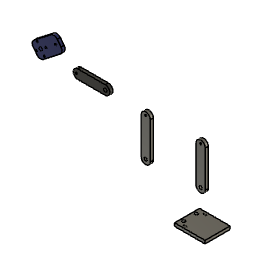
laserCut v11 (Autodesk Fusion 360 design; units mm, degrees)
Autodesk Fusion 360 part; units mm, degrees
sketch "Sketch19" plane through (0, 0, 0) normal (0, 1, 0) x (1, 0, 0)
  line L0 (-204.4398, 88.4329) -> (-125.5431, 26.9894)
  line L1 (-125.5431, 26.9894) -> (-94.8213, 66.4377)
  line L2 (-94.8213, 66.4377) -> (-173.7181, 127.8812)
  line L3 (-173.7181, 127.8812) -> (-204.4398, 88.4329)
  circle A0 centre (-185.1341, 105.0849) radius 3
  circle A1 centre (-182.4324, 77.6313) radius 3
  circle A2 centre (-153.5754, 80.5075) radius 3
  circle A3 centre (-158.4486, 108.3847) radius 3
  circle A4 centre (-121.9436, 56.0242) radius 3
  circle A5 centre (-170.5959, 93.1279) radius 5.5
  dimension "d188" = 50
  dimension "d189" = 100
  dimension "d190" = 6
  dimension "d191" = 6
  dimension "d192" = 6
  dimension "d193" = 6
  dimension "d194" = 40
  dimension "d195" = 25
  dimension "d196" = 25
  dimension "d197" = 39
  dimension "d198" = 5
  dimension "d199" = 24
  dimension "d200" = 5
  dimension "d201" = 6
  dimension "d202" = 40
  dimension "d227" = 11
  dimension "d228" = 19.5
  constraint perpendicular L0 L1
  constraint parallel L0 L2
  constraint parallel L1 L3
  measures "d188" distance of L0.start L2.end
  measures "d189" distance of L0.start L0.end
  measures "d190" diameter of A0
  measures "d191" diameter of A1
  measures "d192" diameter of A2
  measures "d193" diameter of A3
  measures "d194" distance of A0.centre A2.centre
  measures "d195" distance of L2 A0.centre
  measures "d196" distance of L2 A2.centre
  measures "d197" distance of A1.centre A3.centre
  measures "d198" distance of L3 A0.centre
  measures "d199" distance of L3 A1.centre
  measures "d200" distance of L0 A1.centre
  measures "d201" diameter of A4
  measures "d202" distance of A2.centre A4.centre
  measures "d227" diameter of A5
  measures "d228" distance of A1.centre A5.centre
extrude "Extrude1" add sketch "Sketch19" along normal mid plane 10 makes body 1 in component "Link 1"
fillet "Fillet2" radius 15 4 edges at (-204.4398, 0, -88.4329) (-125.5431, 0, -26.9894) (-173.7181, 0, -127.8812) (-94.8213, 0, -66.4377) on bodies 1 in component "Link 1"
sketch "Sketch20" plane through (0, 0, 0) normal (0, 1, 0) x (1, 0, 0)
  line L0 (-230, -110) -> (-110, -110)
  line L1 (-110, -110) -> (-110, -80)
  line L2 (-110, -80) -> (-230, -80)
  line L3 (-230, -80) -> (-230, -110)
  circle A0 centre (-220, -95) radius 3
  circle A1 centre (-125, -95) radius 5.5
  dimension "d205" = 120
  dimension "d206" = 30
  dimension "d207" = 6
  dimension "d208" = 15
  dimension "d209" = 10
  dimension "d325" = 11
  dimension "d326" = 15
  constraint horizontal L0
  constraint vertical L1
  constraint horizontal L2
  constraint vertical L3
  measures "d205" distance of L0.start L0.end
  measures "d206" distance of L0.start L2.end
  measures "d207" diameter of A0
  measures "d208" distance of L2 A0.centre
  measures "d209" distance of L3 A0.centre
  measures "d325" diameter of A1
  measures "d326" distance of L1 A1.centre
extrude "Extrude1'" add sketch "Sketch20" along normal mid plane 10 separate body makes body 2 in component "Link 2"
fillet "Fillet1" radius 15 4 edges at (-230, 0, 80) (-230, 0, 110) (-110, 0, 110) (-110, 0, 80) on bodies 2 in component "Link 2"
sketch "Sketch1" plane through (0, 0, 0) normal (0, 1, 0) x (1, 0, 0) in component "MDholder"
  line L0 (70, 30) -> (100, 30)
  line L1 (100, 30) -> (100, 180)
  line L2 (100, 180) -> (70, 180)
  line L3 (70, 180) -> (70, 30)
  circle A0 centre (85, 40) radius 3
  circle A1 centre (85, 165) radius 5
  dimension "d253" = 150
  dimension "d254" = 6
  dimension "d262" = 10
  dimension "d327" = 10
  dimension "d328" = 15
  constraint horizontal L0
  constraint vertical L1
  constraint horizontal L2
  constraint vertical L3
  measures "d253" distance of L0.start L2.end
  measures "d254" diameter of A0
  measures "d262" distance of L0 A0.centre
  measures "d327" diameter of A1
  measures "d328" distance of L2 A1.centre
extrude "Extrude1''" add sketch "Sketch1" along normal blind 10 separate body makes body 3 in component "MDholder"
fillet "Fillet1'" radius 15 4 edges at (100, 5, -30) (100, 5, -180) (70, 5, -180) (70, 5, -30) on bodies 3 in component "MDholder"
sketch "Sketch1 (2)" plane through (0, 0, 0) normal (0, 1, 0) x (1, 0, 0) in component "holder2"
  line L0 (160, 30) -> (190, 30)
  line L1 (190, 30) -> (190, 180)
  line L2 (190, 180) -> (160, 180)
  line L3 (160, 180) -> (160, 30)
  circle A0 centre (175, 40) radius 3
  circle A1 centre (175, 165) radius 5
  dimension "d259" = 30
  dimension "d260" = 150
  dimension "d261" = 6
  dimension "d263" = 10
  dimension "d329" = 10
  dimension "d330" = 15
  constraint horizontal L0
  constraint vertical L1
  constraint horizontal L2
  constraint vertical L3
  measures "d259" distance of L0.start L0.end
  measures "d260" distance of L0.start L2.end
  measures "d261" diameter of A0
  measures "d263" distance of L0 A0.centre
  measures "d329" diameter of A1
  measures "d330" distance of L2 A1.centre
extrude "Extrude1'''" add sketch "Sketch1 (2)" along normal blind 10 separate body makes body 4 in component "holder2"
fillet "Fillet1''" radius 15 4 edges at (190, 5, -30) (190, 5, -180) (160, 5, -30) (160, 5, -180) on bodies 4 in component "holder2"
sketch "Sketch1 (3)" plane through (0, 0, 0) normal (0, 0, 1) x (1, 0, 0) in component "MD"
  line L0 (200, 150) -> (300, 150)
  line L1 (300, 150) -> (300, 68)
  line L2 (300, 68) -> (200, 68)
  line L3 (200, 68) -> (200, 150)
  circle A0 centre (222.5, 76.5) radius 1.75
  circle A1 centre (222.5, 141.5) radius 1.75
  circle A2 centre (230.5, 141.5) radius 1.75
  circle A3 centre (230.5, 76.5) radius 1.75
  circle A4 centre (210, 88) radius 5
  circle A5 centre (210, 130) radius 5
  dimension "d268" = 100
  dimension "d269" = 82
  dimension "d270" = 3.5
  dimension "d271" = 22.5
  dimension "d272" = 8.5
  dimension "d273" = 3.5
  dimension "d274" = 8.5
  dimension "d275" = 3.5
  dimension "d276" = 8
  dimension "d277" = 3.5
  dimension "d278" = 8
  dimension "d320" = 10
  dimension "d321" = 20
  dimension "d322" = 10
  dimension "d323" = 10
  dimension "d324" = 20
  constraint horizontal L0
  constraint vertical L1
  constraint horizontal L2
  constraint vertical L3
  measures "d268" distance of L0.start L0.end
  measures "d269" distance of L0.start L2.end
  measures "d270" diameter of A0
  measures "d271" distance of L3 A0.centre
  measures "d272" distance of L2 A0.centre
  measures "d273" diameter of A1
  measures "d274" distance of L0 A1.centre
  measures "d275" diameter of A2
  measures "d276" distance of A1.centre A2.centre
  measures "d277" diameter of A3
  measures "d278" distance of A0.centre A3.centre
  measures "d320" diameter of A4
  measures "d321" distance of L2 A4.centre
  measures "d322" distance of L3 A4.centre
  measures "d323" diameter of A5
  measures "d324" distance of L0 A5.centre
extrude "Extrude1''''" add sketch "Sketch1 (3)" along normal blind 10 separate body makes body 5 in component "MD"
component "Link 1" placed x (1, 0, 0) y (0, 1, 0) z (0, 0, 1) at (212.1313, 0, 221.8024)
component "Link 2" placed x (1, 0, 0) y (0, 1, 0) z (0, 0, 1) at (378.3601, 0, 22.7349)
component "MDholder" placed x (1, 0, 0) y (0, 1, 0) z (0, 0, 1) at (251.6524, 44.2391, 103.0246)
component "holder2" placed x (1, 0, 0) y (0, 1, 0) z (0, 0, 1) at (339.6785, 46.3297, 110.6376)
component "MD" placed x (1, 0, 0) y (0, 1, 0) z (0, 0, 1) at (316.5214, -109.0758, -119.7935)
